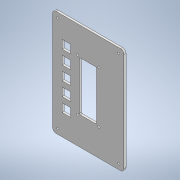
# Autodesk Inventor part: lid
Saved by Autodesk Inventor 2021 (Build 250183000, 183)
## iProperties
Created: 2021-12-13
Part Number: lid
Material: Generic
Document SubType Name: Modeling
Designer: marcin
Density: 1 g/cm^3
Appearance: Default
Author: marcin
Autodesk Inventor part; units mm, degrees
ref_plane "YZ Plane" through (0, 0, 0) normal (1, 0, 0) x (0, 1, 0)
ref_plane "XZ Plane" through (0, 0, 0) normal (0, 1, 0) x (-1, 0, 0)
ref_plane "XY Plane" through (0, 0, 0) normal (0, 0, 1) x (1, 0, 0)
sketch "Sketch2" plane through (0, 0, 0) normal (0, 0, 1) x (1, 0, 0)
  arc A0 (-52, -72) -> (-47, -77) centre (-47, -72) ccw projected
  line L0 (-52, 72) -> (-52, -72) projected
  arc A1 (-47, 77) -> (-52, 72) centre (-47, 72) ccw projected
  line L1 (47, 77) -> (-47, 77) projected
  arc A2 (52, 72) -> (47, 77) centre (47, 72) ccw projected
  line L2 (52, -72) -> (52, 72) projected
  arc A3 (47, -77) -> (52, -72) centre (47, -72) ccw projected
  line L3 (-47, -77) -> (47, -77) projected
  circle A4 centre (44.5, -69.5) radius 1.65 projected
  circle A5 centre (-44.5, -69.5) radius 1.65 projected
  circle A6 centre (-44.5, 69.5) radius 1.65 projected
  circle A7 centre (44.5, 69.5) radius 1.65 projected
  point P0 (0, 0)
extrude "Extrusion2" add sketch "Sketch2" along normal blind 3
sketch "Sketch3" plane through (0, 0, 0) normal (0, 0, -1) x (-1, 0, 0)
  arc A0 (-50, 63) -> (-38, 75) centre (-50, 75) ccw projected
  line L0 (38, 75) -> (-38, 75) projected
  arc A1 (38, 75) -> (50, 63) centre (50, 75) ccw projected
  line L1 (50, -63) -> (50, 63) projected
  line L2 (-50, 63) -> (-50, -63) projected
  arc A2 (-38, -75) -> (-50, -63) centre (-50, -75) ccw projected
  line L3 (-38, -75) -> (38, -75) projected
  arc A3 (50, -63) -> (38, -75) centre (50, -75) ccw projected
  arc A4 (-49.8, 62.8016) -> (-37.8016, 74.8) centre (-50, 75) ccw
  line L4 (-49.8, 62.8016) -> (-49.8, -62.8016)
  arc A5 (-37.8016, -74.8) -> (-49.8, -62.8016) centre (-50, -75) ccw
  line L5 (-37.8016, -74.8) -> (37.8016, -74.8)
  arc A6 (49.8, -62.8016) -> (37.8016, -74.8) centre (50, -75) ccw
  line L6 (49.8, -62.8016) -> (49.8, 62.8016)
  arc A7 (37.8016, 74.8) -> (49.8, 62.8016) centre (50, 75) ccw
  line L7 (37.8016, 74.8) -> (-37.8016, 74.8)
  arc A8 (-47.8, 60.9715) -> (-35.9715, 72.8) centre (-50, 75) ccw
  line L8 (-47.8, 60.9715) -> (-47.8, -60.9715)
  arc A9 (-35.9715, -72.8) -> (-47.8, -60.9715) centre (-50, -75) ccw
  line L9 (-35.9715, -72.8) -> (35.9715, -72.8)
  arc A10 (47.8, -60.9715) -> (35.9715, -72.8) centre (50, -75) ccw
  line L10 (47.8, -60.9715) -> (47.8, 60.9715)
  arc A11 (35.9715, 72.8) -> (47.8, 60.9715) centre (50, 75) ccw
  line L11 (35.9715, 72.8) -> (-35.9715, 72.8)
  point P0 (0, 0)
  dimension "d4" = 0.2
  dimension "d5" = 2
  constraints: 16 end point, 16 point on circle, 8 centre point, 14 other
  measures "d4" radial gap between concentric circles of A0 A4
  measures "d5" radial gap between concentric circles of A4 A8
extrude "Extrusion3" add sketch "Sketch3" along normal blind 2 contours A4 L7 A7 L6 A6 L5 A5 L4
sketch "Sketch4" plane through (0, 0, 3) normal (0, 0, 1) x (1, 0, 0)
  line L0 (11.65, 34.65) -> (11.65, -34.65) projected
  arc A0 (11.65, 34.65) -> (10.65, 35.65) centre (10.65, 34.65) ccw projected
  line L1 (-11.65, 35.65) -> (10.65, 35.65) projected
  arc A1 (-11.65, 35.65) -> (-12.65, 34.65) centre (-11.65, 34.65) ccw projected
  line L2 (-12.65, -34.65) -> (-12.65, 34.65) projected
  arc A2 (-12.65, -34.65) -> (-11.65, -35.65) centre (-11.65, -34.65) ccw projected
  line L3 (10.65, -35.65) -> (-11.65, -35.65) projected
  arc A3 (10.65, -35.65) -> (11.65, -34.65) centre (10.65, -34.65) ccw projected
  line L4 (11.95, -34.65) -> (11.95, 34.65)
  arc A4 (11.95, 34.65) -> (10.65, 35.95) centre (10.65, 34.65) ccw
  line L5 (10.65, 35.95) -> (-11.65, 35.95)
  arc A5 (-11.65, 35.95) -> (-12.95, 34.65) centre (-11.65, 34.65) ccw
  line L6 (-12.95, 34.65) -> (-12.95, -34.65)
  arc A6 (-12.95, -34.65) -> (-11.65, -35.95) centre (-11.65, -34.65) ccw
  line L7 (-11.65, -35.95) -> (10.65, -35.95)
  arc A7 (10.65, -35.95) -> (11.95, -34.65) centre (10.65, -34.65) ccw
  point P0 (0, 0)
  dimension "d10" = 0.3
  constraints: 8 end point, 8 point on circle, 4 centre point, 7 other
  measures "d10" distance between parallel lines of L0 L4
extrude "Extrusion4" cut sketch "Sketch4" against normal up to surface (3 mm away) contours L0 A3 L3 A2 L2 A1 L1 A0 | A7 L7 A6 L6 A5 L5 A4 L4
sketch "Sketch5" plane through (0, 0, 0) normal (0, 0, -1) x (-1, 0, 0)
  circle A0 centre (15.5, 37.5) radius 1.5 projected
  circle A1 centre (-15.5, 37.5) radius 1.5 projected
  circle A2 centre (15.5, -37.5) radius 1.5 projected
  circle A3 centre (-15.5, -37.5) radius 1.5 projected
  circle A4 centre (15.5, -37.5) radius 1.7
  circle A5 centre (15.5, 37.5) radius 1.7
  circle A6 centre (-15.5, 37.5) radius 1.7
  circle A7 centre (-15.5, -37.5) radius 1.7
  point P0 (0, 0)
  dimension "d11" = 0.2
  dimension "d12" = 0.2
  dimension "d13" = 0.2
  dimension "d14" = 0.2
  constraints: 4 centre point
  measures "d11" radial gap between concentric circles of A2 A4
  measures "d12" radial gap between concentric circles of A0 A5
  measures "d13" radial gap between concentric circles of A1 A6
  measures "d14" radial gap between concentric circles of A3 A7
extrude "Extrusion5" cut sketch "Sketch5" against normal up to surface (3 mm away) contours A0 | A1 | A2 | A3 | A4 | A5 | A6 | A7
sketch "Sketch6" plane through (0, 0, 3) normal (0, 0, 1) x (1, 0, 0)
  line L0 (-25.9, 6.1) -> (-38.1, 6.1)
  line L1 (-38.1, 6.1) -> (-38.1, -6.1)
  line L2 (-38.1, -6.1) -> (-25.9, -6.1)
  line L3 (-25.9, -6.1) -> (-25.9, 6.1)
  line L4 (-25.9, 6.1) -> (-38.1, -6.1) construction
  line L5 (-38.1, 6.1) -> (-25.9, -6.1) construction
  line L6 (-52, 72) -> (-52, -72) projected
  line L7 (47, 77) -> (-47, 77) projected
  line L8 (52, -72) -> (52, 72) projected
  line L9 (52, 0) -> (-52, 0)
  point P0 (0, 0)
  point P1 (-32, 0)
  dimension "d17" = 12.2
  dimension "d18" = 12.2
  dimension "d19" = 20
  constraints: 14 end point, 4 midpoint, 2 parallel, 1 horizontal, 1 perpendicular, 1 point on line
  measures "d17" distance of L2.end L1.end
  measures "d18" distance between parallel lines of L0 L2
  measures "d19" distance from line of L6 point (-32, 0)
extrude "Extrusion6" cut sketch "Sketch6" against normal up to surface (3 mm away)
pattern_linear "Rectangular Pattern1" count 3 spacing 20 along (0, -1, 0) count 3 spacing 20 along (0, 1, 0) of "Extrusion6"
body "Solid2"
